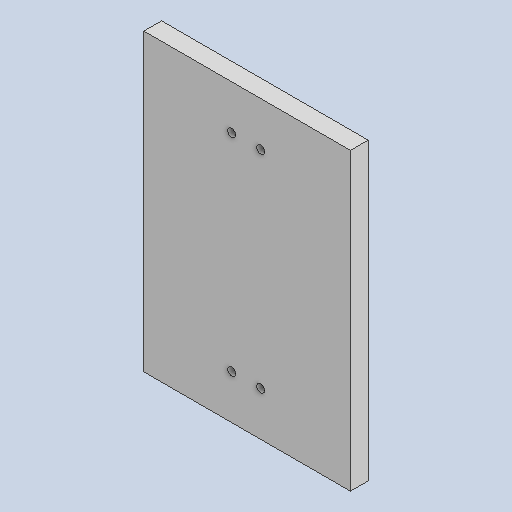
# Autodesk Inventor part: _foot
Saved by Autodesk Inventor 2024.3 (Build 283343000, 343)
## iProperties
Created: 2024-09-05
Part Number: _foot
Material: 일반
Document SubType Name: Modeling
Designer: gretc
Density: 1 g/cm^3
Appearance: 기본값
Author: gretc
Autodesk Inventor part; units mm, degrees
ref_plane "YZ Plane" through (0, 0, 0) normal (1, 0, 0) x (0, 1, 0)
ref_plane "XZ Plane" through (0, 0, 0) normal (0, 1, 0) x (-1, 0, 0)
ref_plane "XY Plane" through (0, 0, 0) normal (0, 0, 1) x (1, 0, 0)
ref_plane "작업 평면1" through (0, -70.02, 0.4347) normal (0, 0, 1) x (1, 0, 0)
sketch "스케치1" plane through (0, -70.02, 0.4347) normal (0, 0, 1) x (1, 0, 0)
  circle A0 centre (18.4, 3) radius 1.35 projected
  circle A1 centre (8.5755, 3) radius 1.35 projected
  line L0 (0, 0) -> (27.6, 0) projected
  line L1 (27.6, 0) -> (27.6, 6) projected
  line L2 (0, 6) -> (27.6, 6) projected
  line L3 (0, 0) -> (0, 6) projected
  circle A2 centre (18.4, 73.02) radius 1.35 projected
  circle A3 centre (8.5755, 73.02) radius 1.35 projected
  line L4 (0, 70.02) -> (27.6, 70.02) projected
  line L5 (27.6, 70.02) -> (27.6, 76.02) projected
  line L6 (0, 76.02) -> (27.6, 76.02) projected
  line L7 (0, 70.02) -> (0, 76.02) projected
  line L8 (13.8, 70.02) -> (13.8, 0)
  line L9 (13.8, 70.02) -> (13.8, 38)
  line L10 (-21.2, -12) -> (-21.2, 88)
  line L11 (-21.2, 88) -> (48.8, 88)
  line L12 (48.8, 88) -> (48.8, -12)
  line L13 (48.8, -12) -> (-21.2, -12)
  line L14 (-21.2, -12) -> (48.8, 88) construction
  line L15 (-21.2, 88) -> (48.8, -12) construction
  point P0 (13.8, 6)
  dimension "d0" = 32.02
  dimension "d1" = 100
  dimension "d2" = 70
  constraints: 16 end point, 5 midpoint, 2 parallel, 2 point on line, 1 perpendicular
  measures "d0" distance of L8.start L9.end
  measures "d1" distance of L10.start L10.end
  measures "d2" distance of L10.end L11.end
extrude "돌출2" add sketch "스케치1" along normal blind 6 contours L3 L2 L8 L0 | L8 L2 L1 L0 | L7 L6 L5 L4 | L10 L11 L12 L13
